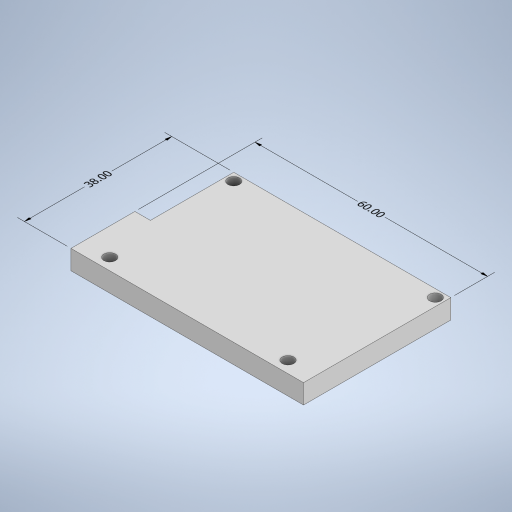
# Autodesk Inventor part: PiBed
Saved by Autodesk Inventor 2024 (Build 280153000, 153)
## iProperties
Created: 2023-05-12
Part Number: PiBed
Material: Generic
Document SubType Name: Modeling
Designer: User
Density: 1 g/cm^3
Appearance: Default
Author: User
Autodesk Inventor part; units mm, degrees
ref_plane "YZ Plane" through (0, 0, 0) normal (1, 0, 0) x (0, 1, 0)
ref_plane "XZ Plane" through (0, 0, 0) normal (0, 1, 0) x (-1, 0, 0)
ref_plane "XY Plane" through (0, 0, 0) normal (0, 0, 1) x (1, 0, 0)
sketch "Sketch2" plane through (0, 0, 0) normal (0, 1, 0) x (-1, 0, 0)
  line L0 (0, 0) -> (-60, 0)
  line L1 (-60, 0) -> (-60, -38)
  line L2 (-60, -38) -> (0, -38)
  line L3 (0, -38) -> (0, 0)
  dimension "d2" = 60
  dimension "d3" = 38
  constraints: 8 end point, 2 parallel, 1 horizontal, 1 perpendicular
  measures "d2" distance of L2.end L1.end
  measures "d3" distance of L1.end L0.end
extrude "Extrusion1" add sketch "Sketch2" along normal blind 5
sketch "Sketch3" plane through (0, 0, 0) normal (0, -1, 0) x (1, 0, 0)
  line L0 (55, -32) -> (5, -32)
  line L1 (5, -32) -> (5, -12)
  line L2 (5, -12) -> (55, -12)
  line L3 (55, -12) -> (55, -32)
  line L4 (60, -38) -> (0, -38) projected
  line L5 (60, 0) -> (60, -38) projected
  point P0 (0, 0)
  dimension "d6" = 50
  dimension "d7" = 20
  dimension "d8" = 6
  dimension "d9" = 5
  constraints: 8 end point, 2 parallel, 1 horizontal, 1 perpendicular
  measures "d6" distance of L1.end L2.end
  measures "d7" distance of L0.end L1.end
  measures "d8" distance between parallel lines of L4 L0
  measures "d9" distance between parallel lines of L5 L3
extrude "Extrusion2" cut sketch "Sketch3" against normal blind 2
sketch "Sketch5" plane through (0, 0, 0) normal (0, -1, 0) x (1, 0, 0)
  circle A0 centre (58, -36) radius 1.5
  line L0 (60, 0) -> (60, -38) projected
  line L1 (60, -38) -> (0, -38) projected
  line L2 (0, -38) -> (0, 0) projected
  dimension "d14" = 3
  dimension "d15" = 2
  dimension "d16" = 2
  constraints: 1 centre point
  measures "d14" diameter of A0
  measures "d15" distance from line of L0 A0.centre
  measures "d16" distance from line of L1 A0.centre
extrude "Extrusion3" cut sketch "Sketch5" against normal blind 5
sketch "Sketch6" plane through (0, 0, 0) normal (0, -1, 0) x (1, 0, 0)
  circle A0 centre (53, -3) radius 1.5
  line L0 (60, 0) -> (60, -38) projected
  line L1 (0, 0) -> (60, 0) projected
  circle A1 centre (7, -3) radius 1.5
  line L2 (0, -38) -> (0, 0) projected
  dimension "d22" = 3
  dimension "d23" = 7
  dimension "d24" = 3
  dimension "d25" = 3
  dimension "d26" = 7
  dimension "d27" = 3
  constraints: 2 centre point
  measures "d22" diameter of A0
  measures "d23" distance from line of L0 A0.centre
  measures "d24" distance from line of L1 A0.centre
  measures "d25" diameter of A1
  measures "d26" distance from line of L2 A1.centre
  measures "d27" distance from line of L1 A1.centre
extrude "Extrusion4" cut sketch "Sketch6" against normal blind 5
sketch "Sketch7" plane through (0, 5, 0) normal (0, 1, 0) x (1, 0, 0)
  line L0 (0, 38) -> (0, 0) projected
  line L1 (0, 38) -> (4, 38)
  line L2 (4, 38) -> (4, 16.5)
  line L3 (4, 16.5) -> (0, 16.5)
  line L4 (0, 16.5) -> (0, 38)
  dimension "d36" = 4
  dimension "d37" = 21.5
  constraints: 8 end point, 2 parallel, 1 horizontal, 1 perpendicular
  measures "d36" distance of L2.end L3.end
  measures "d37" distance of L1.end L2.end
extrude "Extrusion5" cut sketch "Sketch7" against normal blind 10
sketch "Sketch8" plane through (0, 5, 0) normal (0, 1, 0) x (1, 0, 0)
  circle A0 centre (6, 36) radius 1.5
  line L0 (4, 38) -> (4, 16.5) projected
  line L1 (60, 38) -> (4, 38) projected
  point P0 (0, 0)
  dimension "d40" = 3
  dimension "d41" = 2
  dimension "d42" = 2
  constraints: 1 centre point
  measures "d40" diameter of A0
  measures "d41" distance from line of L0 A0.centre
  measures "d42" distance from line of L1 A0.centre
extrude "Extrusion6" cut sketch "Sketch8" against normal blind 10
body "Solid1"
